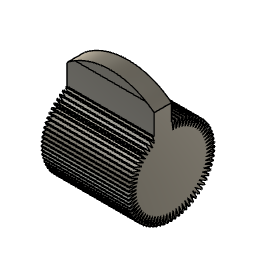
Separate Jig (Autodesk Fusion 360 design; units mm, degrees)
Autodesk Fusion 360 part; units mm, degrees
sketch "Sketch1" plane through (0, 0, 0) normal (1, 0, 0) x (0, 1, 0)
  circle A0 centre (0, 0) radius 25.4
  line L0 (-1.143, 25.3743) -> (1.143, 25.3743)
  line L1 (-1.143, 25.3743) -> (-0.381, 31.4692)
  line L2 (1.143, 25.3743) -> (0.381, 31.4692)
  line L3 (0.381, 31.4692) -> (-0.381, 31.4692)
  line L4 (0, 0) -> (0, 62.9384) construction
  line L5 (0, 0) -> (40.6449, 0) construction
  line L6 (0, 0) -> (16.3268, 19.4575)
  line L7 (0, 0) -> (25.4, 0) construction
  dimension "d1" = 50.8
  dimension "d3" = 0.762
  dimension "d13" = 50
  dimension "d20" = 25.4
  constraint coincident A0.centre L4.start
  constraint coincident A0 L0.start
  constraint coincident A0 L0.end
  constraint horizontal L0
  constraint horizontal L3
  constraint perpendicular L3 L4
  constraint midpoint L3 L4
  constraint horizontal L5
  constraint horizontal L7
  measures "d1" diameter of A0
  measures "d3" distance of L1.end L2.end
  measures "d13" angle of L6 L7
  measures "d20" distance of A0.centre L6.end
extrude "Extrude1" add sketch "Sketch1" along normal blind 63.5 contours A0 L0 picked at (14.1202, -1.7453) makes body 1
extrude "Extrude2" add sketch "Sketch1" along normal blind 63.5 separate body contours A0 L1 L2 L3 makes body 2
pattern_circular "C-Pattern1" count 72 over 360 about axis through (63.5, 0, 0) along (1, 0, 0) of bodies 2 makes body 3 at (21.1667, -3.2742, 27.2241) makes body 4 at (42.3333, -5.6345, 26.8352) makes body 5 at (42.3333, -7.9519, 26.242) makes body 6 at (21.1667, -10.2088, 25.4491) makes body 7 at (42.3333, -12.3879, 24.4625) makes body 8 at (21.1667, -14.4729, 23.2897) makes body 9 at (42.3333, -16.4476, 21.9397) makes body 10 at (21.1667, -18.2972, 20.4227) makes body 11 at (21.1667, -20.0075, 18.7503) makes body 12 at (21.1667, -21.5656, 16.9352) makes body 13 at (21.1667, -22.9595, 14.9912) makes body 14 at (21.1667, -24.1787, 12.9331) makes body 15 at (42.3333, -25.2139, 10.7765) makes body 16 at (21.1667, -26.0572, 8.538) makes body 17 at (21.1667, -26.7022, 6.2345) makes body 18 at (21.1667, -27.1439, 3.8835) makes body 19 at (21.1667, -27.3791, 1.503) makes body 20 at (42.3333, -27.4059, -0.889) makes body 21 at (42.3333, -27.2241, -3.2742) makes body 22 at (42.3333, -26.8352, -5.6345) makes body 23 at (42.3333, -26.242, -7.9519) makes body 24 at (21.1667, -25.4491, -10.2088) makes body 25 at (42.3333, -24.4625, -12.3879) makes body 26 at (42.3333, -23.2897, -14.4729) makes body 27 at (21.1667, -21.9397, -16.4476) makes body 28 at (42.3333, -20.4227, -18.2972) makes body 29 at (21.1667, -18.7503, -20.0075) makes body 30 at (42.3333, -16.9352, -21.5656) makes body 31 at (21.1667, -14.9912, -22.9595) makes body 32 at (21.1667, -12.9331, -24.1787) makes body 33 at (42.3333, -10.7765, -25.2139) makes body 34 at (21.1667, -8.538, -26.0572) makes body 35 at (21.1667, -6.2345, -26.7022) makes body 36 at (42.3333, -3.8835, -27.1439) makes body 37 at (42.3333, -1.503, -27.3791) makes body 38 at (42.3333, 0.889, -27.4059) makes body 39 at (21.1667, 3.2742, -27.2241) makes body 40 at (42.3333, 5.6345, -26.8352) makes body 41 at (42.3333, 7.9519, -26.242) makes body 42 at (21.1667, 10.2088, -25.4491) makes body 43 at (42.3333, 12.3879, -24.4625) makes body 44 at (21.1667, 14.4729, -23.2897) makes body 45 at (21.1667, 16.4476, -21.9397) makes body 46 at (21.1667, 18.2972, -20.4227) makes body 47 at (42.3333, 20.0075, -18.7503) makes body 48 at (42.3333, 21.5656, -16.9352) makes body 49 at (42.3333, 22.9595, -14.9912) makes body 50 at (21.1667, 24.1787, -12.9331) makes body 51 at (21.1667, 25.2139, -10.7765) makes body 52 at (42.3333, 26.0572, -8.538) makes body 53 at (21.1667, 26.7022, -6.2345) makes body 54 at (42.3333, 27.1439, -3.8835) makes body 55 at (21.1667, 27.3791, -1.503) makes body 56 at (42.3333, 27.4059, 0.889) makes body 57 at (21.1667, 27.2241, 3.2742) makes body 58 at (42.3333, 26.8352, 5.6345) makes body 59 at (21.1667, 26.242, 7.9519) makes body 60 at (42.3333, 25.4491, 10.2088) makes body 61 at (21.1667, 24.4625, 12.3879) makes body 62 at (21.1667, 23.2897, 14.4729) makes body 63 at (42.3333, 21.9397, 16.4476) makes body 64 at (21.1667, 20.4227, 18.2972) makes body 65 at (21.1667, 18.7503, 20.0075) makes body 66 at (21.1667, 16.9352, 21.5656) makes body 67 at (21.1667, 14.9912, 22.9595) makes body 68 at (21.1667, 12.9331, 24.1787) makes body 69 at (21.1667, 10.7765, 25.2139) makes body 70 at (21.1667, 8.538, 26.0572) makes body 71 at (21.1667, 6.2345, 26.7022) makes body 72 at (42.3333, 3.8835, 27.1439) makes body 73 at (21.1667, 1.503, 27.3791)
sketch "Sketch2" plane through (63.5, 0, 0) normal (1, 0, 0) x (0, 1, 0)
  arc A0 (-1.143, 25.3743) -> (1.143, 25.3743) centre (0, 0) ccw
  line L0 (1.143, 25.3743) -> (-1.143, 25.3743)
  line L1 (0, 0) -> (25.4, 0) construction
  line L2 (-12.7, 21.997) -> (0, 21.997)
  line L3 (0, 21.997) -> (0, 47.397)
  line L4 (0, 47.397) -> (-12.7, 47.397)
  line L5 (-12.7, 47.397) -> (-12.7, 21.997)
  dimension "d17" = 25.4
  constraint horizontal L1
  constraint coincident A0.centre L1.start
  constraint coincident A0 L2.start
  constraint perpendicular L2 L3
  constraint perpendicular L3 L4
  measures "d17" distance of L2.end L3.end
extrude "Extrude3" add sketch "Sketch2" against normal blind 63.5 contours A0 L0 L2 L3 | A0 L0 L3 L4 L5 picked at (-1.7688, 24.1426) bodies 1 9 10 11 12 13 14 15 16 17 18 19 20 21 22 23 24 25 26 27 28 29 30 31 32 33 34 35 36 37 38 39 40 41 42 43 44 45 46 47 48 49 50 51 52 53 54 55 56 57 58 59 60 61 62 63 64 65 66 67 68 69 70 71 72 73 2 3 4 5 6 7 8
sketch "Sketch4" plane through (0, 0, 0) normal (0, 1, 0) x (-1, 0, 0)
  line L0 (-63.5, 31.4692) -> (0, 31.4692)
  line L1 (0, 31.4692) -> (0, 47.397)
  line L2 (-63.5, 47.397) -> (-63.5, 31.4692)
  arc A0 (15.0645, 36.5279) -> (-78.5645, 36.5279) centre (-31.75, 3.748) ccw
  arc A1 (9.8629, 32.8857) -> (-73.3629, 32.8857) centre (-31.75, 3.748) ccw
  line L3 (15.0645, 36.5279) -> (-31.75, 3.748)
  line L4 (-31.75, 3.748) -> (-78.5645, 36.5279)
  arc A2 (12.4637, 34.7068) -> (-75.9637, 34.7068) centre (-31.75, 3.748) ccw
  dimension "d35" = 6.35
  dimension "d37" = 50.8
  dimension "d42" = 3.175
  constraint coincident A0.centre A1.centre
  constraint coincident A1.start L3
  constraint coincident A1.end L4
  constraint coincident L1.end A2
  constraint coincident L2.start A2
  measures "d35" distance of A0.end A1.end
  measures "d37" radius of A1
extrude "Extrude4" add sketch "Sketch4" against normal blind 254 separate body contours L2 A1 L4 A2 | L1 L2 A1 A2 | L1 A1 L3 A2 | A0 L3 L4 A2 makes body 74
extrude "Extrude5" add sketch "Sketch4" against normal blind 12.7 contours L0 L1 L2 A1 bodies 1 74
sketch "Sketch5" plane through (63.5, 0, 0) normal (1, 0, 0) x (0, 1, 0)
  line L0 (-12.7, 43.4037) -> (-12.7, 28.2771)
  line L1 (-12.7, 28.2771) -> (-12.9542, 28.6818)
  line L2 (-12.9542, 28.6818) -> (-13.6448, 28.3598)
  line L3 (-13.6448, 28.3598) -> (-12.7, 25.4301)
  line L4 (-12.7, 25.4301) -> (-12.7, 23.8709)
  line L5 (-12.7, 23.8709) -> (-15.4046, 27.4436)
  line L6 (-15.4046, 27.4436) -> (-16.0646, 27.0626)
  line L7 (-16.0646, 27.0626) -> (-13.677, 21.4033)
  arc A0 (-13.677, 21.4033) -> (1.143, 25.3743) centre (0, 0) ccw
  line L8 (1.143, 25.3743) -> (0, 25.3743)
  line L9 (0, 25.3743) -> (0, 25.4)
  arc A1 (1.143, 25.3743) -> (0, 25.4) centre (0, 0) ccw
  line L10 (1.143, 25.3743) -> (0.381, 31.4692)
  line L11 (0.381, 31.4692) -> (0, 31.4692)
  line L12 (0, 31.4692) -> (0, 43.4037)
  line L13 (0, 43.4037) -> (-12.7, 43.4037)
  circle A2 centre (0, 0) radius 25.654
  dimension "d47" = 51.308
  constraint concentric A0 A2
  measures "d47" diameter of A2
extrude "Extrude6" add sketch "Sketch5" against normal blind 63.5 contours L7 A0 L10 A2 | L8 L9 A1 | L7 A0 L10 A2 bodies 1 9 10 11 12 13 14 15 16 17 18 19 20 21 22 23 24 25 26 27 28 29 30 31 32 33 34 35 36 37 38 39 40 41 42 43 44 45 46 47 48 49 50 51 52 53 54 55 56 57 58 59 60 61 62 63 64 65 66 67 68 69 70 71 72 73
extrude "Extrude7" cut sketch "Sketch4" against normal blind 342.9 contours L2 A1 L4 A2 | L1 L2 A1 A2 | L1 A1 L3 A2 | A0 L3 L4 A2 bodies 1
equation "w = 0.09 in"
equation "d3 = w / 3"
equation "d42 = ( 0.25 / 2 ) * 1 in"
